Autodesk Fusion 360 part; units mm, degrees
(part 3 of 3)
  point P1444 (32, 17.3205)
  point P1445 (-16, 28)
  point P1446 (-63, 19.3397)
  point P1447 (-48, 28)
  point P1448 (-48, 28)
  point P1449 (32, 17.3205)
  point P1450 (-33, 19.3397)
  point P1451 (33, 19.3397)
  point P1452 (-33, 19.3397)
  point P1453 (-33, 19.3397)
  point P1454 (-48, 28)
  point P1455 (-16, 28)
  point P1456 (-31, 19.3397)
  point P1457 (-1, 19.3397)
  point P1458 (32, 17.3205)
  point P1459 (-16, 28)
  point P1460 (-16, 28)
  point P1461 (-32, 17.3205)
  point P1462 (16, 28)
  point P1463 (-16, 28)
  point P1464 (-16, 28)
  point P1465 (16, 28)
  point P1466 (-31, 19.3397)
  point P1467 (-48, 28)
  point P1468 (-63, 19.3397)
  point P1469 (63, 19.3397)
  point P1470 (0, 17.3205)
  point P1471 (-33, 19.3397)
  point P1472 (-63, 19.3397)
  point P1473 (-16, 28)
  point P1474 (31, 19.3397)
  point P1475 (-48, 28)
  point P1476 (-1, 19.3397)
  point P1477 (-32, 17.3205)
  point P1478 (31, 19.3397)
  point P1479 (16, 28)
  point P1480 (0, 17.3205)
  point P1481 (-33, 19.3397)
  point P1482 (-31, 19.3397)
  point P1483 (-16, 28)
  point P1484 (-63, 19.3397)
  point P1485 (-48, 28)
  point P1486 (-48, 28)
  point P1487 (63, 19.3397)
  point P1488 (-48, 28)
  point P1489 (16, 28)
  point P1490 (-48, 28)
  point P1491 (-48, 28)
  point P1492 (1, 19.3397)
  point P1493 (-48, 28)
  point P1494 (-64, 17.3205)
  point P1495 (-31, 19.3397)
  point P1496 (-48, 28)
  point P1497 (-33, 19.3397)
  point P1498 (-48, 28)
  point P1499 (-48, 28)
  point P1500 (16, 28)
  point P1501 (-63, 19.3397)
  point P1502 (-1, 19.3397)
  point P1503 (16, 28)
  point P1504 (16, 28)
  point P1505 (-48, 28)
  point P1506 (-16, 28)
  point P1507 (1, 19.3397)
  point P1508 (-33, 19.3397)
  point P1509 (63, 19.3397)
  point P1510 (-31, 19.3397)
  point P1511 (1, 19.3397)
  point P1512 (31, 19.3397)
  point P1513 (-63, 19.3397)
  point P1514 (-33, 19.3397)
  point P1515 (-48, 28)
  point P1516 (31, 19.3397)
  point P1517 (-1, 19.3397)
  point P1518 (1, 19.3397)
  point P1519 (-48, 28)
  point P1520 (-48, 28)
  point P1521 (-48, 28)
  point P1522 (16, 28)
  point P1523 (-48, 28)
  point P1524 (-63, 19.3397)
  point P1525 (-48, 28)
  point P1526 (-63, 19.3397)
  point P1527 (64, 17.3205)
  point P1528 (16, 28)
  point P1529 (-16, 28)
  point P1530 (16, 28)
  point P1531 (31, 19.3397)
  point P1532 (-16, 28)
  point P1533 (-31, 19.3397)
  point P1534 (1, 19.3397)
  point P1535 (16, 28)
  point P1536 (-48, 28)
  point P1537 (-32, 0)
  point P1538 (-31, 19.3397)
  point P1539 (-16, 28)
  point P1540 (-16, 28)
  point P1541 (-16, 28)
  point P1542 (-32, 0)
  point P1543 (16, 28)
  point P1544 (16, 28)
  point P1545 (64, 17.3205)
  point P1546 (64, 17.3205)
  point P1547 (-16, 28)
  point P1548 (-16, 28)
  point P1549 (-16, 28)
  point P1550 (-1, 19.3397)
  point P1551 (-1, 19.3397)
  point P1552 (-64, 17.3205)
  point P1553 (-64, 17.3205)
  point P1554 (-32, 0)
  point P1555 (33, 19.3397)
  point P1556 (33, 19.3397)
  point P1557 (-64, 0)
  point P1558 (-16, 28)
  point P1559 (-32, 0)
  point P1560 (31, 19.3397)
  point P1561 (-32, 0)
  point P1562 (16, 28)
  point P1563 (-16, 28)
  point P1564 (31, 19.3397)
  point P1565 (-48, 28)
  point P1566 (16, 28)
  point P1567 (-64, 17.3205)
  point P1568 (-16, 28)
  point P1569 (16, 28)
  point P1570 (64, 17.3205)
  point P1571 (-48, 28)
  point P1572 (32, 0)
  point P1573 (32, 0)
  point P1574 (-32, 0)
  point P1575 (32, 0)
  point P1576 (32, -17.3205)
  point P1577 (0, -17.3205)
  point P1578 (-32, 0)
  point P1579 (32, 0)
  point P1580 (32, 0)
  point P1581 (0, -17.3205)
  point P1582 (32, 0)
  point P1583 (32, -17.3205)
  point P1584 (-64, 0)
  point P1585 (-47, -8.6603)
  point P1586 (32, 0)
  point P1587 (32, 0)
  point P1588 (32, 0)
  point P1589 (-32, 0)
  point P1590 (64, 0)
  point P1591 (32, 0)
  point P1592 (-64, 0)
  point P1593 (17, -8.6603)
  point P1594 (15, -8.6603)
  point P1595 (-15, -8.6603)
  point P1596 (-32, 0)
  point P1597 (-64, 0)
  point P1598 (-32, 0)
  point P1599 (47, -8.6603)
  point P1600 (-32, 0)
  point P1601 (-32, 0)
  point P1602 (-17, -8.6603)
  point P1603 (32, 0)
  point P1604 (32, 0)
  point P1605 (32, -17.3205)
  point P1606 (31, 19.3397)
  point P1607 (31, 19.3397)
  point P1608 (-64, 17.3205)
  point P1609 (33, 19.3397)
  point P1610 (64, 17.3205)
  point P1611 (33, 19.3397)
  point P1612 (-64, 17.3205)
  point P1613 (-64, 17.3205)
  point P1614 (-64, 0)
  point P1615 (-49, -8.6603)
  point P1616 (-47, -8.6603)
  point P1617 (-64, 0)
  point P1618 (-32, -17.3205)
  point P1619 (-64, 0)
  point P1620 (64, 0)
  point P1621 (64, 0)
  point P1622 (-64, 0)
  point P1623 (64, 0)
  point P1624 (-49, -8.6603)
  point P1625 (79, -8.6603)
  point P1626 (-64, 0)
  point P1627 (64, 0)
  point P1628 (64, 0)
  point P1629 (17, -8.6603)
  point P1630 (15, -8.6603)
  point P1631 (-49, -8.6603)
  point P1632 (0, -17.3205)
  point P1633 (-79, -8.6603)
  point P1634 (47, -8.6603)
  point P1635 (-47, -8.6603)
  point P1636 (64, 0)
  point P1637 (49, -8.6603)
  point P1638 (-15, -8.6603)
  point P1639 (-17, -8.6603)
  point P1640 (-64, -17.3205)
  point P1641 (-47, -8.6603)
  point P1642 (32, -17.3205)
  point P1643 (0, -17.3205)
  point P1644 (49, -8.6603)
  point P1645 (32, -17.3205)
  point P1646 (-64, -17.3205)
  point P1647 (32, -17.3205)
  point P1648 (47, -8.6603)
  point P1649 (17, -8.6603)
  point P1650 (15, -8.6603)
  point P1651 (-17, -8.6603)
  point P1652 (-47, -8.6603)
  point P1653 (33, -19.3397)
  point P1654 (-79, -8.6603)
  point P1655 (0, -17.3205)
  point P1656 (-15, -8.6603)
  point P1657 (-47, -8.6603)
  point P1658 (-32, -17.3205)
  point P1659 (79, -8.6603)
  point P1660 (-49, -8.6603)
  point P1661 (0, -17.3205)
  point P1662 (-64, -17.3205)
  point P1663 (-47, -8.6603)
  point P1664 (-64, -17.3205)
  point P1665 (0, -17.3205)
  point P1666 (-64, -17.3205)
  point P1667 (0, -17.3205)
  point P1668 (33, -19.3397)
  point P1669 (33, -19.3397)
  point P1670 (-47, -8.6603)
  point P1671 (-49, -8.6603)
  point P1672 (-49, -8.6603)
  point P1673 (-64, -17.3205)
  point P1674 (0, -17.3205)
  point P1675 (-49, -8.6603)
  point P1676 (32, -17.3205)
  point P1677 (32, 17.3205)
  point P1678 (-1, 19.3397)
  point P1679 (1, 19.3397)
  point P1680 (0, 17.3205)
  point P1681 (32, 17.3205)
  point P1682 (-47, -8.6603)
  point P1683 (-49, -8.6603)
  point P1684 (-31, 19.3397)
  point P1685 (-32, 17.3205)
  point P1686 (32, 17.3205)
  point P1687 (0, 17.3205)
  point P1688 (32, 17.3205)
  point P1689 (-64, 17.3205)
  point P1690 (64, 17.3205)
  point P1691 (79, -8.6603)
  point P1692 (-32, 17.3205)
  point P1693 (-31, 19.3397)
  point P1694 (-32, 17.3205)
  point P1695 (-49, -8.6603)
  point P1696 (-31, 19.3397)
  point P1697 (63, 19.3397)
  point P1698 (31, 19.3397)
  point P1699 (-1, 19.3397)
  point P1700 (-32, 17.3205)
  point P1701 (-32, -17.3205)
  point P1702 (49, -8.6603)
  point P1703 (-1, 19.3397)
  point P1704 (33, 19.3397)
  point P1705 (-64, 17.3205)
  point P1706 (-31, 19.3397)
  point P1707 (-79, -8.6603)
  point P1708 (33, 19.3397)
  point P1709 (1, 19.3397)
  point P1710 (31, 19.3397)
  point P1711 (0, 17.3205)
  point P1712 (64, 17.3205)
  point P1713 (-32, 17.3205)
  point P1714 (1, 19.3397)
  point P1715 (31, 19.3397)
  point P1716 (31, 19.3397)
  point P1717 (-1, 19.3397)
  point P1718 (-1, 19.3397)
  point P1719 (-1, 19.3397)
  point P1720 (-31, 19.3397)
  point P1721 (-33, 19.3397)
  point P1722 (-33, 19.3397)
  point P1723 (-31, 19.3397)
  point P1724 (-32, 17.3205)
  point P1725 (-63, 19.3397)
  point P1726 (1, 19.3397)
  point P1727 (1, 19.3397)
  point P1728 (-63, 19.3397)
  point P1729 (-33, 19.3397)
  point P1730 (-33, 19.3397)
  point P1731 (-31, 19.3397)
  point P1732 (32, 17.3205)
  point P1733 (-31, 19.3397)
  point P1734 (-1, 19.3397)
  point P1735 (0, 17.3205)
  point P1736 (63, 19.3397)
  point P1737 (33, 19.3397)
  point P1738 (31, 19.3397)
  point P1739 (-63, 19.3397)
  point P1740 (-64, 17.3205)
  point P1741 (63, 19.3397)
  point P1742 (-33, 19.3397)
  point P1743 (0, 17.3205)
  point P1744 (-64, 17.3205)
  point P1745 (-63, 19.3397)
  point P1746 (-63, 19.3397)
  point P1747 (31, 19.3397)
  point P1748 (33, 19.3397)
  point P1749 (-1, 19.3397)
  point P1750 (63, 19.3397)
  point P1751 (1, 19.3397)
  point P1752 (-31, 19.3397)
  point P1753 (-63, 19.3397)
  point P1754 (1, 19.3397)
  point P1755 (-33, 19.3397)
  point P1756 (-63, 19.3397)
  point P1757 (-33, 19.3397)
  point P1758 (-63, 19.3397)
  point P1759 (32, 17.3205)
  point P1760 (-31, 19.3397)
  point P1761 (31, 19.3397)
  point P1762 (31, 19.3397)
  point P1763 (-33, 19.3397)
  point P1764 (1, 19.3397)
  point P1765 (1, 19.3397)
  point P1766 (0, 17.3205)
  point P1767 (-33, 19.3397)
  point P1768 (1, 19.3397)
  point P1769 (64, 17.3205)
  point P1770 (-1, 19.3397)
  point P1771 (64, 17.3205)
  point P1772 (32, 17.3205)
  point P1773 (32, 17.3205)
  point P1774 (33, 19.3397)
  point P1775 (-33, 19.3397)
  point P1776 (-1, 19.3397)
  point P1777 (-32, 17.3205)
  point P1778 (-63, 19.3397)
  point P1779 (31, 19.3397)
  point P1780 (-31, 19.3397)
  point P1781 (63, 19.3397)
  point P1782 (-63, 19.3397)
  point P1783 (31, 19.3397)
  point P1784 (1, 19.3397)
  point P1785 (1, 19.3397)
  point P1786 (64, 17.3205)
  point P1787 (-63, 19.3397)
  point P1788 (31, 19.3397)
  point P1789 (0, 17.3205)
  point P1790 (1, 19.3397)
  point P1791 (1, 19.3397)
  point P1792 (-33, 19.3397)
  point P1793 (-31, 19.3397)
  point P1794 (1, 19.3397)
  point P1795 (-1, 19.3397)
  point P1796 (64, 17.3205)
  point P1797 (-63, 19.3397)
  point P1798 (-33, 19.3397)
  point P1799 (-33, 19.3397)
  point P1800 (0, 17.3205)
  point P1801 (-64, 17.3205)
  point P1802 (63, 19.3397)
  point P1803 (31, 19.3397)
  point P1804 (31, 19.3397)
  point P1805 (-1, 19.3397)
  point P1806 (-1, 19.3397)
  point P1807 (64, 17.3205)
  point P1808 (-33, 19.3397)
  point P1809 (-63, 19.3397)
  point P1810 (-31, 19.3397)
  point P1811 (-1, 19.3397)
  point P1812 (-32, 17.3205)
  point P1813 (-31, 19.3397)
  point P1814 (-1, 19.3397)
  point P1815 (-33, 19.3397)
  point P1816 (-63, 19.3397)
  point P1817 (-63, 19.3397)
  point P1818 (63, 19.3397)
  point P1819 (-31, 19.3397)
  dimension "d17" = 140
  dimension "d18" = 140
  dimension "d19" = 120
  dimension "d22" = 2
  constraint horizontal L0
  constraint vertical L1
  constraint horizontal L2
  constraint vertical L3
  constraint coincident A0.centre A1.centre
  constraint coincident P1604 P1603
  constraint coincident P1601 P1600
  constraint coincident P1626 P1622
  constraint coincident P1636 P1628
  constraint coincident P1252 P1250
  constraint coincident P1254 P1241
  constraint coincident P1256 P1255
  constraint coincident P384 P381
  constraint coincident P383 P382
  constraint coincident P378 P377
  constraint coincident P516 P512
  constraint coincident P522 P521
  constraint coincident P308 P307
  constraint coincident P277 P275
  constraint coincident P286 P277
  constraint coincident P286 P275
  constraint coincident P311 P310
  constraint horizontal L249
  constraint coincident P1568 P1563
  constraint coincident P1569 P1566
  constraint coincident P1571 P1565
  measures "d17" distance of L0.start L0.end
  measures "d18" distance of L0.start L2.end
  measures "d19" diameter of A0
extrude "Extrude7" add sketch "Sketch3" along normal blind 40 contours A0 L39 L42 L691 L808 L826 L832 L1153 L1189 L1199 L1227 L1234 L1235 A1 | A0 L36 L39 L42 L309 L497 L518 L695 L699 L708 L709 L808 L826 L890 L891 L892 L893 L1189 L1227 L1234 L1235 L1296 L1297 L1301 L1304 A1 | A0 L1384 L1388 A1 | A0 L1382 L1384 A1 | A0 L677 L1382 A1 | A0 L36 L94 L96 L97 L100 L284 L287 L292 L300 L309 L440 L445 L449 L450 L457 L461 L469 L480 L497 L518 L695 L699 L708 L709 L781 L833 L835 L837 L840 L841 L844 L850 L852 L853 L858 L861 L862 L866 L879 L882 L890 L891 L892 L893 L916 L924 L926 L940 L948 L965 L977 L978 L983 L986 L993 L997 L1001 L1021 L1029 L1032 L1033 L1036 L1041 L1043 L1045 L1062 L1073 L1081 L1085 L1110 L1112 L1115 L1124 L1126 L1269 L1293 L1296 L1297 L1301 L1304 A1 | A0 L34 L35 L36 L39 L42 L45 L46 L48 L49 L52 L94 L96 L97 L99 L100 L101 L104 L105 L106 L108 L110 L111 L112 L113 L114 L115 L116 L119 L122 L124 L130 L133 L136 L137 L141 L144 L147 L150 L151 L155 L156 L160 L162 L168 L169 L172 L176 L181 L193 L199 L201 L203 L205 L217 L223 L225 L228 L237 L245 L247 L248 L254 L256 L270 L271 L276 L280 L281 L284 L287 L288 L292 L295 L300 L303 L304 L308 L309 L312 L321 L326 L331 L332 L333 L334 L335 L337 L338 L345 L348 L349 L350 L352 L357 L359 L362 L366 L370 L382 L383 L384 L388 L390 L392 L395 L396 L404 L405 L407 L409 L412 L415 L418 L420 L426 L428 L429 L430 L434 L437 L440 L443 L444 L445 L446 L448 L449 L450 L455 L456 L457 L460 L461 L463 L464 L466 L468 L469 L472 L475 L476 L477 L480 L482 L487 L488 L490 L495 L497 L500 L502 L504 L507 L509 L510 L518 L519 L520 L531 L534 L536 L542 L549 L551 L552 L554 L558 L560 L584 L589 L591 L592 L595 L612 L631 L632 L634 L635 L646 L654 L661 L662 L663 L669 L670 L671 L674 L675 L677 L682 L684 L685 L690 L691 L694 L695 L698 L699 L706 L708 L709 L710 L715 L728 L737 L740 L742 L748 L753 L757 L761 L768 L772 L774 L778 L781 L782 L808 L819 L826 L832 L833 L834 L835 L837 L839 L840 L841 L843 L844 L845 L846 L847 L850 L852 L853 L854 L856 L857 L858 L859 L860 L861 L862 L863 L866 L868 L869 L870 L871 L872 L879 L880 L882 L890 L891 L892 L893 L911 L913 L916 L919 L922 L924 L925 L926 L931 L932 L936 L937 L940 L946 L948 L951 L965 L969 L972 L975 L977 L978 L982 L983 L986 L990 L991 L993 L996 L997 L1000 L1001 L1002 L1005 L1008 L1013 L1021 L1025 L1029 L1032 L1033 L1036 L1040 L1041 L1043 L1045 L1046 L1048 L1056 L1060 L1061 L1062 L1064 L1065 L1068 L1071 L1073 L1074 L1075 L1078 L1080 L1081 L1082 L1083 L1085 L1089 L1092 L1094 L1098 L1100 L1102 L1104 L1106 L1107 L1109 L1110 L1111 L1112 L1113 L1114 L1115 L1119 L1121 L1122 L1124 L1126 L1134 L1146 L1147 L1149 L1153 L1164 L1171 L1173 L1175 L1185 L1188 L1189 L1191 L1199 L1201 L1202 L1205 L1211 L1212 L1213 L1226 L1227 L1232 L1234 L1235 L1244 L1245 L1254 L1269 L1271 L1272 L1291 L1292 L1293 L1296 L1297 L1301 L1304 L1309 L1311 L1318 L1321 L1335 L1336 L1339 L1343 L1354 L1365 L1366 L1369 L1373 L1379 L1382 L1383 L1384 L1386 L1387 L1388 L1391 L1393 L1394 L1395 | A0 L677 L691 L832 L1153 L1199 A1 | A0 L1388 L1391 A1 | A0 L94 L96 L97 L100 L110 L113 L205 L284 L287 L292 L300 L332 L382 L404 L405 L426 L440 L445 L449 L450 L457 L461 L469 L480 L781 L833 L835 L837 L840 L841 L844 L850 L852 L853 L858 L861 L862 L866 L879 L882 L916 L924 L926 L940 L948 L965 L977 L978 L983 L986 L993 L997 L1001 L1021 L1029 L1032 L1033 L1036 L1041 L1043 L1045 L1062 L1073 L1081 L1085 L1110 L1112 L1115 L1124 L1126 L1269 L1293 L1373 A1 | A0 L1391 L1395 A1 | A0 L110 L113 L147 L156 L199 L205 L217 L332 L382 L384 L390 L404 L405 L407 L426 L429 L1373 A1 | A0 L1393 L1395 A1 | A0 L122 L147 L156 L168 L199 L217 L335 L338 L383 L384 L390 L407 L415 L420 L428 L429 A1 | A0 L682 L1393 A1 | A0 L122 L130 L133 L168 L245 L254 L335 L338 L383 L388 L395 L415 L418 L420 L428 L437 A1 | A0 L682 L684 L860 L1173 L1185 A1 | A0 L130 L133 L136 L169 L245 L254 L303 L321 L388 L395 L418 L437 L468 L495 L500 L558 A1 | A0 L48 L49 L52 L201 L446 L482 L728 L748 L768 L782 L854 L859 L911 L913 L931 L951 L969 L972 L1002 L1008 L1201 L1202 L1244 L1254 A1 | A0 L49 L52 L684 L854 L859 L860 L1173 L1185 L1201 L1202 L1244 L1254 A1 | A0 L124 L136 L169 L176 L303 L304 L321 L333 L448 L468 L495 L500 L507 L520 L558 L560 A1 | A0 L48 L116 L201 L334 L444 L446 L482 L536 L715 L728 L740 L742 L748 L768 L778 L782 L911 L913 L919 L931 L937 L951 L969 L972 L1002 L1008 L1068 L1092 L1098 L1100 L1107 L1119 A1 | A0 L124 L155 L176 L181 L270 L280 L304 L333 L448 L464 L502 L507 L520 L552 L554 L560 A1 | A0 L116 L119 L193 L334 L444 L455 L490 L536 L715 L740 L742 L778 L919 L937 L1068 L1092 L1098 L1100 L1107 L1119 L1379 A1 | A0 L119 L155 L181 L193 L270 L280 L455 L464 L490 L502 L552 L554 L1379 A1 makes body 1
extrude "Extrude6" add sketch "Sketch3" along normal blind 5 separate body contours L0 L3 L39 L41 L42 L43 L587 L588 L593 L604 L605 L607 L609 L610 L611 L613 L621 L630 L636 L660 L664 L673 L676 L677 L691 L795 L808 L826 L827 L832 L1153 L1157 L1172 L1189 L1199 L1214 L1221 L1227 L1234 L1235 L1380 L1381 L1382 A1 | L0 L1380 L1381 L1382 L1384 L1385 A1 | L3 L36 L39 L40 L41 L42 L43 L233 L309 L496 L497 L514 L518 L695 L699 L704 L707 L708 L709 L795 L799 L808 L822 L826 L827 L888 L889 L890 L891 L892 L893 L1157 L1172 L1189 L1214 L1221 L1227 L1234 L1235 L1295 L1296 L1297 L1299 L1301 L1302 L1303 L1304 L1306 L1307 A1 | L0 L1384 L1385 L1388 L1389 A1 | L2 L3 L36 L40 L94 L95 L96 L97 L98 L100 L102 L103 L107 L109 L110 L113 L120 L134 L140 L143 L145 L147 L148 L149 L154 L156 L157 L161 L163 L194 L199 L205 L210 L217 L233 L249 L262 L272 L273 L284 L287 L292 L293 L294 L296 L300 L302 L309 L311 L318 L319 L320 L323 L324 L328 L330 L332 L382 L384 L386 L390 L399 L404 L405 L406 L407 L419 L426 L429 L440 L445 L449 L450 L453 L457 L461 L469 L479 L480 L493 L496 L497 L513 L514 L515 L518 L524 L525 L527 L533 L548 L550 L562 L563 L695 L699 L704 L707 L708 L709 L781 L799 L822 L833 L835 L837 L840 L841 L844 L850 L852 L853 L858 L861 L862 L866 L879 L882 L886 L887 L888 L889 L890 L891 L892 L893 L894 L895 L896 L897 L898 L899 L900 L901 L902 L903 L904 L905 L906 L907 L916 L924 L926 L940 L948 L965 L977 L978 L983 L986 L993 L997 L1001 L1021 L1029 L1032 L1033 L1036 L1041 L1043 L1045 L1062 L1073 L1081 L1085 L1110 L1112 L1115 L1124 L1126 L1269 L1293 L1295 L1296 L1297 L1299 L1301 L1302 L1303 L1304 L1306 L1307 L1372 L1373 A1 | L0 L1388 L1389 L1390 L1391 A1 | A0 L39 L42 L691 L808 L826 L832 L1153 L1189 L1199 L1227 L1234 L1235 A1 | A0 L36 L39 L42 L309 L497 L518 L695 L699 L708 L709 L808 L826 L890 L891 L892 L893 L1189 L1227 L1234 L1235 L1296 L1297 L1301 L1304 A1 | L0 L1390 L1391 L1395 L1396 A1 | A0 L1384 L1388 A1 | A0 L1382 L1384 A1 | A0 L677 L1382 A1 | A0 L36 L94 L96 L97 L100 L284 L287 L292 L300 L309 L440 L445 L449 L450 L457 L461 L469 L480 L497 L518 L695 L699 L708 L709 L781 L833 L835 L837 L840 L841 L844 L850 L852 L853 L858 L861 L862 L866 L879 L882 L890 L891 L892 L893 L916 L924 L926 L940 L948 L965 L977 L978 L983 L986 L993 L997 L1001 L1021 L1029 L1032 L1033 L1036 L1041 L1043 L1045 L1062 L1073 L1081 L1085 L1110 L1112 L1115 L1124 L1126 L1269 L1293 L1296 L1297 L1301 L1304 A1 | A0 L677 L691 L832 L1153 L1199 A1 | L587 L588 L593 L604 L605 L607 L609 L610 L611 L613 L621 L630 L636 L660 L664 L673 L676 L677 L691 L832 L1153 L1199 A1 | L0 L1392 L1393 L1395 L1396 L1397 A1 | A0 L1388 L1391 A1 | L2 L140 L143 L145 L148 L154 L157 L161 L163 L249 L262 L272 L273 L294 L311 L319 L328 L330 | L94 L95 L96 L97 L98 L100 L102 L103 L107 L109 L110 L113 L194 L205 L210 L284 L287 L292 L296 L300 L302 L318 L320 L332 L382 L386 L399 L404 L405 L406 L419 L426 L440 L445 L449 L450 L457 L461 L469 L480 L493 L513 L524 L525 L533 L548 L550 L562 L781 L833 L835 L837 L840 L841 L844 L850 L852 L853 L858 L861 L862 L866 L879 L882 L886 L887 L894 L895 L896 L897 L898 L899 L900 L901 L902 L903 L904 L905 L906 L907 L916 L924 L926 L940 L948 L965 L977 L978 L983 L986 L993 L997 L1001 L1021 L1029 L1032 L1033 L1036 L1041 L1043 L1045 L1062 L1073 L1081 L1085 L1110 L1112 L1115 L1124 L1126 L1269 L1293 L1372 L1373 A1 | A0 L94 L96 L97 L100 L110 L113 L205 L284 L287 L292 L300 L332 L382 L404 L405 L426 L440 L445 L449 L450 L457 L461 L469 L480 L781 L833 L835 L837 L840 L841 L844 L850 L852 L853 L858 L861 L862 L866 L879 L882 L916 L924 L926 L940 L948 L965 L977 L978 L983 L986 L993 L997 L1001 L1021 L1029 L1032 L1033 L1036 L1041 L1043 L1045 L1062 L1073 L1081 L1085 L1110 L1112 L1115 L1124 L1126 L1269 L1293 L1373 A1 | L0 L1 L49 L50 L52 L53 L572 L574 L643 L656 L682 L683 L684 L828 L854 L855 L859 L860 L1173 L1185 L1201 L1202 L1228 L1233 L1238 L1239 L1244 L1254 L1392 L1393 L1397 A1 | A0 L1391 L1395 A1 | A0 L110 L113 L147 L156 L199 L205 L217 L332 L382 L384 L390 L404 L405 L407 L426 L429 L1373 A1 | A0 L1393 L1395 A1 | L2 L120 L122 L134 L147 L149 L156 L168 L171 L199 L217 L224 L249 L293 L323 L324 L335 L338 L383 L384 L390 L407 L415 L420 L428 L429 L453 L479 L515 L527 L563 L564 A1 | A0 L122 L147 L156 L168 L199 L217 L335 L338 L383 L384 L390 L407 L415 L420 L428 L429 A1 | L1 L48 L49 L50 L51 L52 L53 L201 L317 L391 L446 L462 L482 L726 L728 L748 L765 L768 L771 L782 L783 L828 L854 L855 L859 L911 L913 L929 L931 L944 L945 L951 L961 L969 L972 L994 L1002 L1008 L1012 L1014 L1019 L1201 L1202 L1228 L1233 L1238 L1239 L1244 L1254 A1 | A0 L682 L1393 A1 | L2 L122 L125 L126 L129 L130 L133 L135 L158 L166 L168 L171 L173 L174 L175 L192 L209 L221 L224 L226 L245 L249 L254 L255 L257 L258 L259 L335 L336 L338 L383 L388 L395 L415 L418 L420 L428 L437 L564 L565 A1 | A0 L122 L130 L133 L168 L245 L254 L335 L338 L383 L388 L395 L415 L418 L420 L428 L437 A1 | L1 L2 L48 L51 L116 L117 L118 L119 L123 L128 L131 L132 L142 L153 L155 L159 L179 L181 L183 L187 L189 L190 L193 L201 L204 L214 L215 L234 L249 L260 L263 L265 L266 L267 L270 L274 L277 L280 L285 L317 L322 L325 L334 L387 L391 L394 L442 L444 L446 L455 L462 L464 L467 L471 L482 L484 L485 L490 L492 L494 L498 L499 L501 L502 L503 L508 L512 L517 L532 L536 L552 L553 L554 L555 L556 L568 L569 L715 L726 L728 L740 L742 L748 L765 L768 L771 L778 L782 L783 L911 L913 L919 L929 L931 L937 L944 L945 L951 L961 L969 L972 L994 L1002 L1008 L1012 L1014 L1019 L1068 L1092 L1098 L1100 L1107 L1119 L1141 L1231 L1250 L1342 L1378 L1379 A1 | A0 L682 L684 L860 L1173 L1185 A1 | L572 L574 L643 L656 L682 L683 L684 L860 L1173 L1185 A1 | L2 L126 L129 L135 L158 L166 L173 L174 L175 L192 L209 L221 L226 L249 L257 L258 L259 L336 | L2 L125 L130 L133 L136 L169 L170 L245 L246 L249 L254 L255 L303 L321 L388 L395 L418 L437 L468 L495 L500 L558 L565 L566 A1 | A0 L130 L133 L136 L169 L245 L254 L303 L321 L388 L395 L418 L437 L468 L495 L500 L558 A1 | L1 L2 L128 L131 L142 L153 L159 L177 L187 L189 L249 L260 L263 L265 L266 L274 L277 L297 L325 L467 L484 L492 L494 L498 L501 L503 L508 L517 L532 L553 L556 L569 L570 | A0 L48 L49 L52 L201 L446 L482 L728 L748 L768 L782 L854 L859 L911 L913 L931 L951 L969 L972 L1002 L1008 L1201 L1202 L1244 L1254 A1 | A0 L49 L52 L684 L854 L859 L860 L1173 L1185 L1201 L1202 L1244 L1254 A1 | L2 L124 L136 L139 L146 L169 L170 L176 L178 L180 L182 L184 L185 L186 L188 L246 L249 L261 L264 L275 L278 L282 L286 L289 L303 L304 L316 L321 L329 L333 L448 L468 L495 L500 L507 L520 L558 L560 L566 L567 A1 | A0 L124 L136 L169 L176 L303 L304 L321 L333 L448 L468 L495 L500 L507 L520 L558 L560 A1 | L1 L2 L177 L249 L297 L570 | A0 L48 L116 L201 L334 L444 L446 L482 L536 L715 L728 L740 L742 L748 L768 L778 L782 L911 L913 L919 L931 L937 L951 L969 L972 L1002 L1008 L1068 L1092 L1098 L1100 L1107 L1119 A1 | L2 L123 L124 L132 L155 L176 L179 L181 L186 L249 L264 L267 L270 L280 L285 L304 L322 L333 L442 L448 L464 L471 L499 L502 L507 L512 L520 L552 L554 L560 L567 L568 A1 | A0 L124 L155 L176 L181 L270 L280 L304 L333 L448 L464 L502 L507 L520 L552 L554 L560 A1 | A0 L116 L119 L193 L334 L444 L455 L490 L536 L715 L740 L742 L778 L919 L937 L1068 L1092 L1098 L1100 L1107 L1119 L1379 A1 | L116 L117 L118 L119 L193 L215 L234 L334 L387 L394 L444 L455 L485 L490 L536 L555 L715 L740 L742 L778 L919 L937 L1068 L1092 L1098 L1100 L1107 L1119 L1141 L1231 L1250 L1342 L1378 L1379 A1 | A0 L119 L155 L181 L193 L270 L280 L455 L464 L490 L502 L552 L554 L1379 A1 | L2 L139 L146 L178 L180 L182 L184 L185 L188 L249 L261 L275 L278 L282 L286 L289 L316 L329 | L2 L183 L190 L204 L214 L249 makes body 2
sketch "Sketch4" plane through (0, 0, 5) normal (0, 0, 1) x (-1, 0, 0)
  circle A0 centre (0, 0) radius 60
  line L0 (70.0229, 70.078) -> (-69.9771, 70.078)
  line L1 (-69.9771, 70.078) -> (-69.9771, -69.922)
  line L2 (-69.9771, -69.922) -> (70.0229, -69.922)
  line L3 (70.0229, -69.922) -> (70.0229, 70.078)
  line L4 (52.5, -52.5) -> (-52.5, -52.5)
  line L5 (-52.5, -52.5) -> (-52.5, 52.5)
  line L6 (-52.5, 52.5) -> (52.5, 52.5)
  line L7 (52.5, 52.5) -> (52.5, -52.5)
  line L8 (52.5, -52.5) -> (-52.5, 52.5) construction
  line L9 (-52.5, -52.5) -> (52.5, 52.5) construction
  dimension "d25" = 105
  dimension "d26" = 105
  constraint horizontal L4
  constraint perpendicular L4 L5
  constraint parallel L4 L6
  constraint parallel L5 L7
  constraint coincident L8 A0.centre
  constraint coincident L9 A0.centre
  constraint coincident A0.centre origin
  measures "d25" distance of L5.end L6.end
  measures "d26" distance of L4.end L5.end
hole "Hole2" at (-52.5, 52.5, 5) at (52.5, 52.5, 5) at (-52.5, -52.5, 5) at (52.5, -52.5, 5) direction (0, 0, -1) diameter 5 depth 5 tip angle 180 bodies 2
